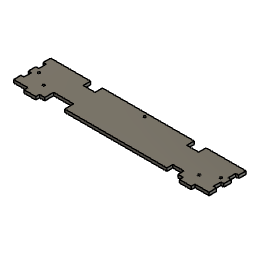
move_base_sidewall_3 (Autodesk Fusion 360 design; units mm, degrees)
Autodesk Fusion 360 part; units mm, degrees
sketch "スケッチ1" plane through (0, 0, 0) normal (0, 1, 0) x (1, 0, 0)
  line L0 (-132, 0) -> (132, 0)
  line L1 (-132, 0) -> (-132, -10)
  line L2 (-132, -10) -> (-128, -10)
  line L3 (-128, -10) -> (-128, -20)
  line L4 (-128, -20) -> (-132, -20)
  line L5 (-132, -20) -> (-132, -30)
  line L6 (-132, -30) -> (-128, -30)
  line L7 (-128, -30) -> (-128, -40)
  line L8 (-128, -40) -> (-132, -40)
  line L9 (-132, -40) -> (-132, -50)
  line L10 (-132, -50) -> (132, -50)
  line L11 (132, 0) -> (132, -10)
  line L12 (132, -10) -> (128, -10)
  line L13 (128, -10) -> (128, -20)
  line L14 (128, -20) -> (132, -20)
  line L15 (132, -20) -> (132, -30)
  line L16 (132, -30) -> (128, -30)
  line L17 (128, -30) -> (128, -40)
  line L18 (128, -40) -> (132, -40)
  line L19 (132, -40) -> (132, -50)
  line L20 (-78, 0) -> (-62, 0)
  line L21 (-62, 0) -> (-62, -10)
  line L22 (-62, -10) -> (-78, -10)
  line L23 (-78, -10) -> (-78, 0)
  line L24 (62, 0) -> (78, 0)
  line L25 (78, 0) -> (78, -10)
  line L26 (78, -10) -> (62, -10)
  line L27 (62, -10) -> (62, 0)
  line L28 (-113, -55) -> (-97, -55)
  line L29 (-97, -55) -> (-97, -50)
  line L30 (-97, -50) -> (-113, -50)
  line L31 (-113, -50) -> (-113, -55)
  line L32 (97, -55) -> (113, -55)
  line L33 (113, -55) -> (113, -50)
  line L34 (113, -50) -> (97, -50)
  line L35 (97, -50) -> (97, -55)
  line L36 (-90, -50) -> (-63, -50)
  line L37 (-63, -50) -> (-63, -38)
  line L38 (-63, -38) -> (-90, -38)
  line L39 (-90, -38) -> (-90, -50)
  line L40 (90, -50) -> (75, -50)
  line L41 (75, -50) -> (75, -42)
  line L42 (75, -42) -> (90, -42)
  line L43 (90, -42) -> (90, -50)
  point P0 (0, -25)
  point P1 (-105, -50)
  point P2 (105, -50)
  dimension "d1" = 264
  dimension "d2" = 10
  dimension "d3" = 10
  dimension "d4" = 10
  dimension "d5" = 10
  dimension "d6" = 10
  dimension "d7" = 4
  dimension "d9" = 4
  dimension "d40" = 62
  dimension "d41" = 16
  dimension "d42" = 10
  dimension "d43" = 62
  dimension "d45" = 5
  dimension "d46" = 16
  dimension "d47" = 105
  dimension "d48" = 105
  dimension "d51" = 63
  dimension "d52" = 27
  dimension "d53" = 12
  dimension "d54" = 75
  dimension "d55" = 15
  dimension "d56" = 8
  constraint horizontal L0
  constraint midpoint origin L0
  constraint perpendicular L0 L1
  constraint perpendicular L1 L2
  constraint perpendicular L0 L3
  constraint perpendicular L3 L4
  constraint perpendicular L4 L5
  constraint perpendicular L3 L6
  constraint perpendicular L6 L7
  constraint perpendicular L7 L8
  constraint perpendicular L8 L9
  constraint perpendicular L9 L10
  constraint collinear L1 L5
  constraint collinear L5 L9
  constraint collinear L3 L7
  constraint perpendicular L0 L11
  constraint perpendicular L11 L12
  constraint perpendicular L0 L13
  constraint perpendicular L13 L14
  constraint perpendicular L14 L15
  constraint perpendicular L13 L16
  constraint perpendicular L14 L17
  constraint perpendicular L13 L18
  constraint perpendicular L18 L19
  constraint collinear L11 L15
  constraint collinear L15 L19
  constraint collinear L13 L17
  constraint collinear L2 L12
  constraint collinear L4 L14
  constraint collinear L6 L16
  constraint collinear L8 L18
  constraint vertical origin P0
  constraint coincident L10.end L19.end
  constraint horizontal L20
  constraint vertical L21
  constraint horizontal L22
  constraint vertical L23
  constraint coincident L0 L20.start
  constraint horizontal L24
  constraint vertical L25
  constraint horizontal L26
  constraint vertical L27
  constraint coincident L0 L24.start
  constraint collinear L22 L26
  constraint equal L22 L26
  constraint horizontal L28
  constraint vertical L29
  constraint horizontal L30
  constraint vertical L31
  constraint horizontal L32
  constraint vertical L33
  constraint horizontal L34
  constraint vertical L35
  constraint midpoint L30 P1
  constraint midpoint L34 P2
  constraint equal L29 L35
  constraint equal L28 L32
  constraint coincident L10 P1
  constraint coincident L10 P2
  constraint horizontal L36
  constraint vertical L37
  constraint horizontal L38
  constraint vertical L39
  constraint coincident L10 L36.start
  constraint horizontal L40
  constraint vertical L41
  constraint horizontal L42
  constraint vertical L43
  constraint coincident L10 L40.start
  measures "d1" distance of L0.start L0.end
  measures "d2" distance of L0.start L1.end
  measures "d3" distance of L2.end L3.end
  measures "d4" distance of L4.end L5.end
  measures "d5" distance of L6.end L7.end
  measures "d6" distance of L8.end L9.end
  measures "d7" distance of L1.end L2.end
  measures "d9" distance of L11.end L12.end
  measures "d40" distance of origin L21
  measures "d41" distance of L20.start L20.end
  measures "d42" distance of L20.end L21.end
  measures "d43" distance of origin L27
  measures "d45" distance of L28.start L30.end
  measures "d46" distance of L28.start L28.end
  measures "d47" horizontal distance of origin P1
  measures "d48" horizontal distance of origin P2
  measures "d51" distance of origin L37
  measures "d52" distance of L37 L39
  measures "d53" distance of L36.end L37.end
  measures "d54" distance of origin L41
  measures "d55" distance of L41 L43
  measures "d56" distance of L40.end L41.end
extrude "押し出し1" add sketch "スケッチ1" along normal blind 4 contours L0 L1 L2 L3 L4 L5 L6 L7 L8 L9 L10 L11 L12 L13 L14 L15 L16 L17 L18 L19 L21 L22 L23 L25 L26 L27 L30 L34 L37 L38 L39 L41 L42 L43 | L10 L28 L29 L30 L31 | L10 L32 L33 L34 L35
sketch "スケッチ2" plane through (0, 4, 0) normal (0, 1, 0) x (-1, 0, 0)
  line L0 (-132, 50) -> (-132, 40)
  line L1 (-132, 40) -> (-128, 40)
  line L2 (-128, 40) -> (-128, 30)
  line L3 (-128, 30) -> (-132, 30)
  line L4 (-132, 30) -> (-132, 20)
  line L5 (-132, 20) -> (-128, 20)
  line L6 (-128, 20) -> (-128, 10)
  line L7 (-128, 10) -> (-132, 10)
  line L8 (-132, 10) -> (-132, 0)
  line L9 (-62, 0) -> (62, 0)
  line L10 (123, 25) -> (-123, 25)
  line L11 (105, 36.5) -> (-105, 36.5)
  line L12 (132, 0) -> (132, 10)
  line L13 (132, 10) -> (128, 10)
  line L14 (128, 10) -> (128, 20)
  line L15 (128, 20) -> (132, 20)
  line L16 (132, 20) -> (132, 30)
  line L17 (132, 30) -> (128, 30)
  line L18 (128, 30) -> (128, 40)
  line L19 (128, 40) -> (132, 40)
  line L20 (132, 40) -> (132, 50)
  line L21 (63, 50) -> (-75, 50)
  line L22 (-78, 0) -> (-78, 10)
  line L23 (-78, 10) -> (-62, 10)
  line L24 (-62, 10) -> (-62, 0)
  line L25 (62, 0) -> (62, 10)
  line L26 (62, 10) -> (78, 10)
  line L27 (78, 10) -> (78, 0)
  line L28 (78, 0) -> (132, 0)
  line L29 (-132, 0) -> (-78, 0)
  line L30 (113, 50) -> (113, 55)
  line L31 (113, 55) -> (97, 55)
  line L32 (97, 55) -> (97, 50)
  line L33 (97, 50) -> (90, 50)
  line L34 (-97, 50) -> (-97, 55)
  line L35 (-97, 55) -> (-113, 55)
  line L36 (-113, 55) -> (-113, 50)
  line L37 (-113, 50) -> (-132, 50)
  line L38 (-75, 50) -> (-75, 42)
  line L39 (-75, 42) -> (-90, 42)
  line L40 (-90, 42) -> (-90, 50)
  line L41 (-90, 50) -> (-97, 50)
  line L42 (132, 50) -> (113, 50)
  line L43 (90, 50) -> (90, 38)
  line L44 (90, 38) -> (63, 38)
  line L45 (63, 38) -> (63, 50)
  point P0 (0, 5)
  dimension "d17" = 25
  dimension "d19" = 5
  dimension "d24" = 105
  dimension "d25" = 105
  dimension "d44" = 5
  dimension "d49" = 13.5
  dimension "d50" = 5
  constraint horizontal L10
  constraint horizontal L11
  constraint vertical origin P0
  measures "d17" distance of origin L10
  measures "d19" distance of L6 L10.end
  measures "d24" horizontal distance of origin L11.start
  measures "d25" horizontal distance of origin L11.end
  measures "d44" distance of origin P0
  measures "d49" distance of L11 L33
  measures "d50" distance of L10.start L14
hole "穴1" at (-123, 4, 25) at (123, 4, 25) at (-105, 4, 36.5) at (105, 4, 36.5) at (0, 4, 5) direction (0, -1, 0) diameter 3.2 end through all
